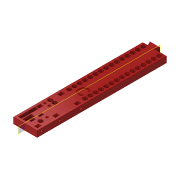
# Autodesk Inventor part: Coupler extension arm short
Saved by Autodesk Inventor 2020 (Build 240168000, 168)
## iProperties
Created: 2019-10-02
Part Number: Coupler extension arm short
Material: Generic
Document SubType Name: Modeling
Designer: ball
Density: 1 g/cm^3
Appearance: Default
Author: ball
Autodesk Inventor part; units mm, degrees
ref_plane "YZ Plane" through (0, 0, 0) normal (1, 0, 0) x (0, 1, 0)
ref_plane "XZ Plane" through (0, 0, 0) normal (0, 1, 0) x (-1, 0, 0)
ref_plane "XY Plane" through (0, 0, 0) normal (0, 0, 1) x (1, 0, 0)
sketch "Sketch1" plane through (0, 0, 0) normal (0, 1, 0) x (-1, 0, 0)
  line L0 (0, 0) -> (35.5, 0)
  line L1 (35.5, 0) -> (35.5, -195)
  line L2 (35.5, -195) -> (0, -195)
  line L3 (0, -195) -> (0, 0)
  dimension "d0" = 35.5
  dimension "d1" = 195
  constraints: 8 end point, 2 parallel, 1 horizontal, 1 perpendicular
  measures "d0" distance of L1.end L2.end
  measures "d1" distance of L0.end L1.end
extrude "BlockShape" add sketch "Sketch1" along normal blind 9
sketch "Sketch3" plane through (0, 0, 0) normal (0, -1, 0) x (1, 0, 0)
  circle A0 centre (-10, -25) radius 3.25 construction
  line L0 (0, 0) -> (-35.5, 0) projected
  line L1 (-35.5, 0) -> (-35.5, -195) projected
  line L2 (-11.6286, -27.8125) -> (-13.25, -24.9958)
  line L3 (-13.25, -24.9958) -> (-11.6214, -22.1833)
  line L4 (-11.6214, -22.1833) -> (-8.3714, -22.1875)
  line L5 (-8.3714, -22.1875) -> (-6.75, -25.0042)
  line L6 (-6.75, -25.0042) -> (-8.3786, -27.8167)
  line L7 (-8.3786, -27.8167) -> (-11.6286, -27.8125)
  line L8 (0, -195) -> (0, 0) projected
  dimension "d15" = 6.5
  dimension "d16" = 25
  dimension "d26" = 10
  constraints: 12 end point, 1 coincident, 16 other
  measures "d16" distance from line of L0 point (-10, -25)
  measures "d26" distance from line of L8 point (-10, -25)
extrude "SlideMountingNutWell1" cut sketch "Sketch3" against normal blind 5
sketch "Sketch5" plane through (0, 9, 0) normal (0, 1, 0) x (1, 0, 0)
  line L0 (0, 0) -> (0, 195) projected
  line L1 (-35.5, 0) -> (0, 0) projected
  circle A0 centre (-10, 25) radius 1.7
  circle A1 centre (-10, 15) radius 1.7
  dimension "d36" = 3.4
  dimension "d37" = 25
  dimension "d137" = 3.4
  dimension "d138" = 15
  constraints: 2 centre point
  measures "d36" diameter of A0
  measures "d37" distance from line of L1 A0.centre
  measures "d137" diameter of A1
  measures "d138" distance from line of L1 A1.centre
extrude "SlideMountingHoles" cut sketch "Sketch5" against normal through all
sketch "Sketch6" plane through (0, 9, 0) normal (0, 1, 0) x (1, 0, 0)
  line L0 (-32.5, 4) -> (-27.7502, 4)
  line L1 (-27.7502, 4) -> (-27.7502, 29.4)
  line L2 (-27.7502, 29.4) -> (-32.5, 29.4)
  line L3 (-32.5, 29.4) -> (-32.5, 4)
  line L4 (-35.5, 0) -> (0, 0) projected
  line L5 (-35.5, 195) -> (-35.5, 0) projected
  line L6 (-25.7502, 4) -> (-21.0002, 4)
  line L7 (-21.0002, 4) -> (-21.0002, 16.7)
  line L8 (-21.0002, 16.7) -> (-25.7502, 16.7)
  line L9 (-25.7502, 16.7) -> (-25.7502, 4)
  line L10 (0, 0) -> (0, 195) construction
  line L11 (-35.5, 195) -> (0, 195) projected
  line L12 (0, 0) -> (-20, 0) construction
  line L13 (-20, 0) -> (-20, 195) construction
  line L14 (-20, 195) -> (0, 195) construction
  line L15 (0, 195) -> (0, 0)
  circle A0 centre (-23.3752, 41.7) radius 1.7
  circle A1 centre (-30.125, 41.7) radius 1.7
  circle A2 centre (-30.125, 49.7) radius 1.7
  circle A3 centre (-23.3752, 49.7) radius 1.7
  dimension "d43" = 4.7498
  dimension "d44" = 25.4
  dimension "d45" = 4
  dimension "d46" = 3
  dimension "d47" = 4.75
  dimension "d48" = 2
  dimension "d49" = 20
  dimension "d50" = 3.4
  dimension "d90" = 3.4
  dimension "d91" = 5.375
  dimension "d92" = 3.4
  dimension "d94" = 3.4
  dimension "d246" = 41.7
  dimension "d247" = 49.7
  dimension "d248" = 41.7
  dimension "d249" = 49.7
  constraints: 24 end point, 6 parallel, 4 centre point, 3 horizontal, 3 perpendicular, 1 point on line
  measures "d43" distance of L2.end L1.end
  measures "d44" distance of L1.end L0.end
  measures "d45" distance between parallel lines of L4 L0
  measures "d46" distance between parallel lines of L5 L3
  measures "d47" distance of L8.end L7.end
  measures "d48" distance between parallel lines of L9 L1
  measures "d49" distance of L13.end L14.end
  measures "d50" diameter of A0
  measures "d90" diameter of A1
  measures "d91" distance from line of L5 A1.centre
  measures "d92" diameter of A2
  measures "d94" diameter of A3
  measures "d246" distance from line of L4 A0.centre
  measures "d247" distance from line of L4 A3.centre
  measures "d248" distance from line of L4 A1.centre
  measures "d249" distance from line of L4 A2.centre
extrude "Shape" cut sketch "Sketch6" against normal through all contours L3 L2 L1 L0 | L9 L8 L7 L6 | A0 | A1 | A2 | A3
sketch "Sketch7" plane through (0, 0, 0) normal (0, -1, 0) x (1, 0, 0)
  circle A0 centre (-23.3752, -41.7) radius 1.7 projected
  circle A1 centre (-23.3752, -41.7) radius 3.25 construction
  line L0 (-23.3752, -38.45) -> (-20.5606, -40.075)
  line L1 (-20.5606, -40.075) -> (-20.5606, -43.325)
  line L2 (-20.5606, -43.325) -> (-23.3752, -44.95)
  line L3 (-23.3752, -44.95) -> (-26.1898, -43.325)
  line L4 (-26.1898, -43.325) -> (-26.1898, -40.075)
  line L5 (-26.1898, -40.075) -> (-23.3752, -38.45)
  line L6 (0, 0) -> (-35.5, 0) projected
  circle A2 centre (-30.125, -41.7) radius 3.25 construction
  line L7 (-35.5, 0) -> (-35.5, -195) projected
  line L8 (-30.1645, -44.9498) -> (-32.9591, -43.2907)
  line L9 (-32.9591, -43.2907) -> (-32.9196, -40.0409)
  line L10 (-32.9196, -40.0409) -> (-30.0855, -38.4502)
  line L11 (-30.0855, -38.4502) -> (-27.2909, -40.1093)
  line L12 (-27.2909, -40.1093) -> (-27.3304, -43.3591)
  line L13 (-27.3304, -43.3591) -> (-30.1645, -44.9498)
  dimension "d88" = 6.5
  dimension "d54" = 6.5
  dimension "d87" = 41.7
  dimension "d89" = 5.375
  constraints: 24 end point, 3 coincident, 1 centre point, 17 other
  measures "d54" diameter of A1
  measures "d87" distance from line of L6 A1.centre
  measures "d89" distance from line of L7 point (-30.125, -41.7)
extrude "TensionNutWells1" cut sketch "Sketch7" against normal blind 5
sketch "Sketch8" plane through (-35.5, 0, -195) normal (-1, 0, 0) x (0, 0, 1)
  circle A0 centre (184.65, 4.5) radius 1.4605
  line L0 (0, 9) -> (195, 9) projected
  line L1 (195, 0) -> (195, 9) projected
  circle A1 centre (171.95, 4.5) radius 1.4605
  dimension "d57" = 2.921
  dimension "d58" = 4.5
  dimension "d59" = 10.35
  dimension "d103" = 2.921
  dimension "d104" = 4.5
  dimension "d105" = 12.7
  constraints: 2 centre point
  measures "d57" diameter of A0
  measures "d58" distance from line of L0 A0.centre
  measures "d59" distance from line of L1 A0.centre
  measures "d103" diameter of A1
  measures "d104" distance from line of L0 A1.centre
  measures "d105" distance of A0.centre A1.centre
hole "PulleyMountingHoles" at (-35.5, 4.5, -10.35) at (-35.5, 4.5, -23.05) direction (1, 0, 0) diameter 2.921 depth 22.5 counterbore diameter 3.4 counterbore depth 1.5
sketch "Sketch9" plane through (-21.0002, 9, -16.7) normal (-1, 0, 0) x (0, 0, 1)
  circle A0 centre (6.35, -4.5) radius 1.4605 projected
  circle A1 centre (6.35, -4.5) radius 2.54
  point P0 (16.7, -9)
  dimension "d67" = 5.08
  constraints: 1 centre point, 1 coincident
  measures "d67" diameter of A1
extrude "PulleyStandoff1" add sketch "Sketch9" along normal blind 0.2032
sketch "Sketch10" plane through (-27.7502, 9, -29.4) normal (-1, 0, 0) x (0, 0, 1)
  circle A0 centre (6.35, -4.5) radius 1.7 projected
  circle A1 centre (6.35, -4.5) radius 2.54
  circle A2 centre (19.05, -4.5) radius 2.54 projected
  circle A3 centre (19.05, -4.5) radius 2.54
  circle A4 centre (19.05, -4.5) radius 1.7
  point P0 (29.4, -9)
  dimension "d70" = 5.08
  dimension "d106" = 3.4
  constraints: 3 centre point, 3 coincident
  measures "d70" diameter of A1
  measures "d106" diameter of A4
extrude "PulleyStandoff3" add sketch "Sketch10" along normal blind 0.2032
sketch "Sketch11" plane through (-25.7502, 9, -4) normal (1, 0, 0) x (0, 0, -1)
  circle A0 centre (6.35, -4.5) radius 1.7 projected
  circle A1 centre (6.35, -4.5) radius 2.54
  point P0 (-4, -9)
  dimension "d73" = 5.08
  constraints: 1 centre point, 1 coincident
  measures "d73" diameter of A1
extrude "PulleyStandoff2" add sketch "Sketch11" along normal blind 0.2032
sketch "Sketch12" plane through (-32.5, 9, -4) normal (1, 0, 0) x (0, 0, -1)
  circle A0 centre (6.35, -4.5) radius 1.7 projected
  circle A1 centre (6.35, -4.5) radius 2.54
  circle A2 centre (19.05, -4.5) radius 1.4605 projected
  circle A3 centre (19.05, -4.5) radius 2.54
  circle A4 centre (19.05, -4.5) radius 1.7
  point P0 (-4, -9)
  dimension "d76" = 5.08
  dimension "d107" = 5.08
  dimension "d108" = 3.4
  constraints: 3 centre point, 3 coincident
  measures "d76" diameter of A1
  measures "d107" diameter of A3
  measures "d108" diameter of A4
extrude "PulleyStandof4" add sketch "Sketch12" along normal blind 0.2032 contours A1 | A3
sketch "Sketch14" plane through (0, 0, -195) normal (0, 0, -1) x (-1, 0, 0)
  circle A0 centre (18, 4.5) radius 2.25
  line L0 (35.5, 0) -> (0, 0) projected
  line L1 (0, 0) -> (0, 9) projected
  dimension "d82" = 4.5
  dimension "d83" = 4.5
  dimension "d84" = 18
  constraints: 1 centre point
  measures "d82" diameter of A0
  measures "d83" distance from line of L0 A0.centre
  measures "d84" distance from line of L1 A0.centre
extrude "4mmShaft" cut sketch "Sketch14" against normal blind 41
sketch "Sketch15" plane through (0, 9, 0) normal (0, 1, 0) x (1, 0, 0)
  circle A0 centre (-30.125, 49.7) radius 1.7 projected
  circle A1 centre (-30.125, 49.7) radius 3.25 construction
  circle A2 centre (-23.3752, 49.7) radius 1.7 projected
  circle A3 centre (-23.3752, 49.7) radius 3.25 construction
  line L0 (-30.125, 52.95) -> (-27.3104, 51.325)
  line L1 (-27.3104, 51.325) -> (-27.3104, 48.075)
  line L2 (-27.3104, 48.075) -> (-30.125, 46.45)
  line L3 (-30.125, 46.45) -> (-32.9396, 48.075)
  line L4 (-32.9396, 48.075) -> (-32.9396, 51.325)
  line L5 (-32.9396, 51.325) -> (-30.125, 52.95)
  line L6 (-23.3752, 52.95) -> (-20.5606, 51.325)
  line L7 (-20.5606, 51.325) -> (-20.5606, 48.075)
  line L8 (-20.5606, 48.075) -> (-23.3752, 46.45)
  line L9 (-23.3752, 46.45) -> (-26.1898, 48.075)
  line L10 (-26.1898, 48.075) -> (-26.1898, 51.325)
  line L11 (-26.1898, 51.325) -> (-23.3752, 52.95)
  point P0 (0, 0)
  dimension "d95" = 6.5
  dimension "d96" = 6.5
  constraints: 24 end point, 4 coincident, 2 vertical alignment, 30 other
extrude "TensionNutWells2" cut sketch "Sketch15" against normal blind 5
ref_plane "PulleyMidPlane1" through (-30.1251, 9, -4) normal (1, 0, 0) x (0, 0, -1)
ref_plane "PulleyMidPlane2" through (-23.3752, 9, -4) normal (1, 0, 0) x (0, 0, -1)
sketch "Sketch26" plane through (-35.5, 0, -195) normal (-1, 0, 0) x (0, 0, 1)
  line L0 (165.6, 9) -> (165.6, 0) construction
  line L1 (156.5498, 0) -> (156.5498, 5) construction
  line L2 (138.824, 0) -> (135.776, 0) construction
  line L3 (5.524, 0) -> (2.476, 0) construction
  circle A0 centre (161.0749, 4.5) radius 1.45 construction
  circle A1 centre (103.213, 4.5) radius 1.45 construction
  line L4 (135.776, 9) -> (135.776, 0) construction
  line L5 (5.524, 9) -> (5.524, 0) construction
  line L6 (0, 9) -> (195, 9) projected
  circle A2 centre (70.65, 4.5) radius 1.45 construction
  circle A3 centre (38.087, 4.5) radius 1.45 construction
  point P0 (195, 0)
  dimension "d192" = 2.9
  dimension "d193" = 2.9
  dimension "d196" = 130.252
  dimension "d197" = 32.563
  dimension "d198" = 4.5
  dimension "d199" = 4.5
  dimension "d202" = 32.563
  dimension "d207" = 9.0502
  dimension "d208" = 4.5251
  constraints: 4 centre point, 3 coincident, 1 horizontal, 4 other
  measures "d192" diameter of A0
  measures "d193" diameter of A1
  measures "d196" distance between parallel lines of L5 L4
  measures "d197" distance from line of L4 A1.centre
  measures "d198" distance from line of L6 A0.centre
  measures "d199" distance from line of L6 A1.centre
  measures "d202" distance of A1.centre A2.centre
  measures "d207" distance between parallel lines of L1 L0
  measures "d208" distance from line of L0 A0.centre
ref_plane "Work Plane3" through (-7.7, 0, 0) normal (1, 0, 0) x (0, 0, -1)
sketch "Sketch27" plane through (-7.7, 0, 0) normal (1, 0, 0) x (0, 0, -1)
  line L0 (195, 9) -> (0, 9) projected
  line L1 (0, 0) -> (0, 9) projected
  circle A0 centre (6.65, 4.5) radius 3.45 construction
  line L2 (6.65, 1.05) -> (3.6622, 2.775)
  line L3 (3.6622, 2.775) -> (3.6622, 9)
  line L4 (9.6378, 9) -> (9.6378, 2.775)
  line L5 (9.6378, 2.775) -> (6.65, 1.05)
  line L6 (3.6622, 9) -> (9.6378, 9)
  circle A1 centre (33.9251, 4.5) radius 3.45 construction
  line L7 (33.9251, 1.05) -> (30.9373, 2.775)
  line L8 (30.9373, 2.775) -> (30.9373, 9)
  line L9 (36.9129, 9) -> (36.9129, 2.775)
  line L10 (36.9129, 2.775) -> (33.9251, 1.05)
  line L11 (30.9373, 9) -> (36.9129, 9)
  circle A2 centre (66, 4.5) radius 3.45 construction
  line L12 (66, 1.05) -> (63.0122, 2.775)
  line L13 (63.0122, 2.775) -> (63.0122, 9)
  line L14 (68.9878, 9) -> (68.9878, 2.775)
  line L15 (68.9878, 2.775) -> (66, 1.05)
  line L16 (63.0122, 9) -> (68.9878, 9)
  dimension "d218" = 6.9
  dimension "d283" = 6.9
  dimension "d288" = 6.9
  dimension "d216" = 4.5
  dimension "d217" = 6.65
  dimension "d281" = 33.9251
  dimension "d282" = 4.5
  dimension "d287" = 66
  constraints: 30 end point, 6 coincident, 3 vertical alignment, 2 point on line, 1 collinear, 24 other
  measures "d216" distance from line of L0 point (6.65, 4.5)
  measures "d217" distance from line of L1 point (6.65, 4.5)
  measures "d281" distance from line of L1 point (33.925, 4.5)
  measures "d282" distance from line of L0 point (33.925, 4.5)
  measures "d287" distance from line of L1 point (66, 4.5)
extrude "SideNutWell" cut sketch "Sketch27" along normal blind 4.4
sketch "Sketch28" plane through (0, 0, 0) normal (1, 0, 0) x (0, 0, -1)
  line L0 (9.6378, 2.775) -> (9.6378, 9) construction
  line L1 (3.6622, 9) -> (3.6622, 2.775) construction
  line L2 (3.6622, 2.775) -> (6.65, 1.05) construction
  line L3 (6.65, 1.05) -> (9.6378, 2.775) construction
  circle A0 centre (6.65, 4.5) radius 1.7
  line L4 (195, 0) -> (0, 0) projected
  circle A1 centre (66, 4.5) radius 1.7
  line L5 (0, 0) -> (0, 9) projected
  circle A2 centre (33.9251, 4.5) radius 1.7
  dimension "d221" = 3.4
  dimension "d222" = 4.5
  dimension "d291" = 3.4
  dimension "d292" = 66
  dimension "d293" = 4.5
  dimension "d295" = 3.4
  dimension "d296" = 33.9251
  dimension "d297" = 4.5
  constraints: 3 centre point
  measures "d221" diameter of A0
  measures "d222" distance from line of L4 A0.centre
  measures "d291" diameter of A1
  measures "d292" distance from line of L5 A1.centre
  measures "d293" distance from line of L4 A1.centre
  measures "d295" diameter of A2
  measures "d296" distance from line of L5 A2.centre
  measures "d297" distance from line of L4 A2.centre
extrude "SideNetWellHole" cut sketch "Sketch28" against normal blind 8.4
ref_plane "Work Plane4" through (-27.8, 0, -195) normal (-1, 0, 0) x (0, 0, 1)
sketch "Sketch30" plane through (-27.8, 0, -195) normal (-1, 0, 0) x (0, 0, 1)
  circle A0 centre (161.0749, 4.5) radius 3.45 construction
  line L0 (165.6, 9) -> (165.6, 0) construction
  line L1 (164.445, 0) -> (155.555, 0) construction
  line L2 (161.0749, 1.05) -> (158.0871, 2.775)
  line L3 (158.0871, 2.775) -> (158.0871, 6.225)
  line L4 (164.0627, 6.225) -> (164.0627, 2.775)
  line L5 (164.0627, 2.775) -> (161.0749, 1.05)
  line L6 (164.0627, 6.225) -> (164.0627, 9)
  line L7 (195, 9) -> (0, 9) projected
  line L8 (158.0871, 6.225) -> (158.0871, 9)
  line L9 (158.0696, 9) -> (158.0696, 3.048) projected
  line L10 (158.0871, 9) -> (164.0627, 9)
  line L11 (195, 0) -> (195, 9) projected
  line L12 (0, 0) -> (195, 0) projected
  circle A1 centre (129, 4.5) radius 3.45 construction
  line L13 (129, 1.05) -> (126.0122, 2.775)
  line L14 (126.0122, 2.775) -> (126.0122, 6.225)
  line L15 (131.9878, 6.225) -> (131.9878, 2.775)
  line L16 (131.9878, 2.775) -> (129, 1.05)
  line L17 (131.9878, 6.225) -> (131.9878, 9)
  line L18 (126.0122, 6.225) -> (126.0122, 9)
  line L19 (126.0122, 9) -> (131.9878, 9)
  point P0 (158.0871, 9)
  point P1 (131.9878, 9)
  point P2 (126.0122, 9)
  dimension "d228" = 6.9
  dimension "d286" = 6.9
  dimension "d229" = 4.5251
  dimension "d230" = 4.5
  dimension "d280" = 33.9251
  dimension "d284" = 66
  dimension "d285" = 4.5
  constraints: 28 end point, 2 coincident, 2 perpendicular, 2 vertical, 2 vertical alignment, 1 parallel, 1 point on line, 20 other
  measures "d229" distance from line of L0 point (161.075, 4.5)
  measures "d230" distance from line of L1 point (161.075, 4.5)
  measures "d280" distance from line of L11 point (161.075, 4.5)
  measures "d284" distance from line of L11 point (129, 4.5)
  measures "d285" distance from line of L12 point (129, 4.5)
extrude "SideNutWell2" cut sketch "Sketch30" along normal blind 4.4
sketch "Sketch31" plane through (-35.5, 0, -195) normal (-1, 0, 0) x (0, 0, 1)
  circle A0 centre (161.0749, 4.5) radius 1.45 construction
  circle A1 centre (161.0749, 4.5) radius 1.7
  circle A2 centre (129, 4.5) radius 1.7
  line L0 (195, 0) -> (195, 9) projected
  dimension "d233" = 3.4
  dimension "d289" = 3.4
  dimension "d290" = 66
  dimension "d294" = 33.9251
  constraints: 2 centre point, 1 coincident
  measures "d233" diameter of A1
  measures "d289" diameter of A2
  measures "d290" distance from line of L0 A2.centre
  measures "d294" distance from line of L0 A0.centre
extrude "SideNutWellHole2" cut sketch "Sketch31" against normal blind 8.4
sketch "Sketch33" plane through (0, 0, 0) normal (0, -1, 0) x (1, 0, 0)
  line L0 (0, -195) -> (-35.5, -195) projected
  line L1 (-27.9958, -195) -> (-19.0042, -195)
  line L2 (-19.0042, -195) -> (-19.0042, -195.254)
  line L3 (-19.0042, -195.254) -> (-27.9958, -195.254) construction
  line L4 (-27.9958, -195.254) -> (-27.9958, -195)
  line L5 (-23.5, -195.254) -> (-23.5, -195) construction
  line L6 (-35.5, 0) -> (-35.5, -195) construction
  line L7 (-27.9958, -195.254) -> (-19.0042, -195.254) construction
  line L8 (-19.0042, -195.254) -> (-19.0042, -201.35) construction
  line L9 (-19.0042, -201.35) -> (-27.9958, -201.35)
  line L10 (-27.9958, -201.35) -> (-27.9958, -195.254) construction
  line L11 (-27.9958, -201.35) -> (-31.0438, -201.35)
  line L12 (-31.0438, -201.35) -> (-27.9958, -195.254)
  line L13 (-19.0042, -201.35) -> (-15.9562, -201.35)
  line L14 (-15.9562, -201.35) -> (-19.0042, -195.254)
  point P0 (0, 0)
  dimension "d237" = 8.9916
  dimension "d238" = 0.254
  dimension "d239" = 12
  dimension "d240" = 8.9916
  dimension "d241" = 6.096
  dimension "d242" = 3.048
  dimension "d243" = 3.048
  constraints: 26 end point, 5 parallel, 2 horizontal, 2 midpoint, 2 perpendicular, 2 point on line
  measures "d237" distance of L2.end L3.end
  measures "d238" distance of L1.end L2.end
  measures "d239" distance between parallel lines of L6 L5
  measures "d240" distance of L8.end L9.end
  measures "d241" distance between parallel lines of L3 L9
  measures "d242" distance from line of L11.end L10
  measures "d243" distance from line of L13.end L8
extrude "Extrusion22" add sketch "Sketch33" against normal up to surface (9 mm away)
sketch "Sketch34" plane through (0, 0, 0) normal (0, -1, 0) x (1, 0, 0)
  circle A0 centre (-5.75, -78) radius 2 construction
  circle A1 centre (-29.75, -78) radius 2 construction
  circle A2 centre (-5.75, -78) radius 1.7
  circle A3 centre (-29.75, -78) radius 1.7
  line L0 (0, -195) -> (0, 0) projected
  circle A4 centre (-5.75, -86) radius 1.7
  circle A5 centre (-29.75, -86) radius 1.7
  circle A6 centre (-5.75, -94) radius 1.7
  circle A7 centre (-29.75, -94) radius 1.7
  circle A8 centre (-5.75, -102) radius 1.7
  circle A9 centre (-29.75, -102) radius 1.7
  circle A10 centre (-5.75, -110) radius 1.7
  circle A11 centre (-29.75, -110) radius 1.7
  circle A12 centre (-5.75, -118) radius 1.7
  circle A13 centre (-29.75, -118) radius 1.7
  circle A14 centre (-5.75, -126) radius 1.7
  circle A15 centre (-29.75, -126) radius 1.7
  circle A16 centre (-5.75, -134) radius 1.7
  circle A17 centre (-29.75, -134) radius 1.7
  circle A18 centre (-5.75, -142) radius 1.7
  circle A19 centre (-29.75, -142) radius 1.7
  circle A20 centre (-5.75, -150) radius 1.7
  circle A21 centre (-29.75, -150) radius 1.7
  circle A22 centre (-5.75, -158) radius 1.7
  circle A23 centre (-29.75, -158) radius 1.7
  circle A24 centre (-5.75, -166) radius 1.7
  circle A25 centre (-29.75, -166) radius 1.7
  circle A26 centre (-5.75, -174) radius 1.7
  circle A27 centre (-29.75, -174) radius 1.7
  circle A28 centre (-5.75, -182) radius 1.7
  circle A29 centre (-29.75, -182) radius 1.7
  circle A30 centre (-5.75, -190) radius 1.7
  circle A31 centre (-29.75, -190) radius 1.7
  dimension "d250" = 3.4
  dimension "d251" = 3.4
  dimension "d254" = 8
  constraints: 32 centre point, 2 coincident, 1 vertical, 60 other
  measures "d250" diameter of A2
  measures "d251" diameter of A3
  measures "d254" distance of A2.centre A4.centre
extrude "Extrusion23" cut sketch "Sketch34" against normal through all
sketch "Sketch35" plane through (0, 9, 0) normal (0, 1, 0) x (1, 0, 0)
  circle A0 centre (-29.75, 78) radius 1.7 construction
  circle A1 centre (-29.75, 78) radius 3.25 construction
  circle A2 centre (-5.75, 78) radius 1.7 construction
  circle A3 centre (-5.75, 78) radius 3.25 construction
  line L0 (-26.5, 78) -> (-28.125, 75.1854)
  line L1 (-28.125, 75.1854) -> (-31.375, 75.1854)
  line L2 (-31.375, 75.1854) -> (-33, 78)
  line L3 (-33, 78) -> (-31.375, 80.8146)
  line L4 (-31.375, 80.8146) -> (-28.125, 80.8146)
  line L5 (-28.125, 80.8146) -> (-26.5, 78)
  line L6 (-2.5, 78) -> (-4.125, 75.1854)
  line L7 (-4.125, 75.1854) -> (-7.375, 75.1854)
  line L8 (-7.375, 75.1854) -> (-9, 78)
  line L9 (-9, 78) -> (-7.375, 80.8146)
  line L10 (-7.375, 80.8146) -> (-4.125, 80.8146)
  line L11 (-4.125, 80.8146) -> (-2.5, 78)
  line L12 (-35.5, 195) -> (-35.5, 0) construction
  line L13 (-28.125, 83.1854) -> (-31.375, 83.1854)
  line L14 (-31.375, 83.1854) -> (-33, 86)
  line L15 (-26.5, 86) -> (-28.125, 83.1854)
  circle A4 centre (-29.75, 86) radius 3.25 construction
  line L16 (-33, 86) -> (-31.375, 88.8146)
  line L17 (-31.375, 88.8146) -> (-28.125, 88.8146)
  line L18 (-28.125, 88.8146) -> (-26.5, 86)
  line L19 (-7.375, 83.1854) -> (-9, 86)
  line L20 (-4.125, 83.1854) -> (-7.375, 83.1854)
  line L21 (-2.5, 86) -> (-4.125, 83.1854)
  line L22 (-9, 86) -> (-7.375, 88.8146)
  line L23 (-4.125, 88.8146) -> (-2.5, 86)
  circle A5 centre (-5.75, 86) radius 3.25 construction
  line L24 (-7.375, 88.8146) -> (-4.125, 88.8146)
  line L25 (-28.125, 91.1854) -> (-31.375, 91.1854)
  line L26 (-31.375, 91.1854) -> (-33, 94)
  line L27 (-26.5, 94) -> (-28.125, 91.1854)
  circle A6 centre (-29.75, 94) radius 3.25 construction
  line L28 (-33, 94) -> (-31.375, 96.8146)
  line L29 (-31.375, 96.8146) -> (-28.125, 96.8146)
  line L30 (-28.125, 96.8146) -> (-26.5, 94)
  line L31 (-7.375, 91.1854) -> (-9, 94)
  line L32 (-4.125, 91.1854) -> (-7.375, 91.1854)
  line L33 (-2.5, 94) -> (-4.125, 91.1854)
  line L34 (-9, 94) -> (-7.375, 96.8146)
  line L35 (-4.125, 96.8146) -> (-2.5, 94)
  circle A7 centre (-5.75, 94) radius 3.25 construction
  line L36 (-7.375, 96.8146) -> (-4.125, 96.8146)
  line L37 (-28.125, 99.1854) -> (-31.375, 99.1854)
  line L38 (-31.375, 99.1854) -> (-33, 102)
  line L39 (-26.5, 102) -> (-28.125, 99.1854)
  circle A8 centre (-29.75, 102) radius 3.25 construction
  line L40 (-33, 102) -> (-31.375, 104.8146)
  line L41 (-31.375, 104.8146) -> (-28.125, 104.8146)
  line L42 (-28.125, 104.8146) -> (-26.5, 102)
  line L43 (-7.375, 99.1854) -> (-9, 102)
  line L44 (-4.125, 99.1854) -> (-7.375, 99.1854)
  line L45 (-2.5, 102) -> (-4.125, 99.1854)
  line L46 (-9, 102) -> (-7.375, 104.8146)
  line L47 (-4.125, 104.8146) -> (-2.5, 102)
  circle A9 centre (-5.75, 102) radius 3.25 construction
  line L48 (-7.375, 104.8146) -> (-4.125, 104.8146)
  line L49 (-28.125, 107.1854) -> (-31.375, 107.1854)
  line L50 (-31.375, 107.1854) -> (-33, 110)
  line L51 (-26.5, 110) -> (-28.125, 107.1854)
  circle A10 centre (-29.75, 110) radius 3.25 construction
  line L52 (-33, 110) -> (-31.375, 112.8146)
  line L53 (-31.375, 112.8146) -> (-28.125, 112.8146)
  line L54 (-28.125, 112.8146) -> (-26.5, 110)
  line L55 (-7.375, 107.1854) -> (-9, 110)
  line L56 (-4.125, 107.1854) -> (-7.375, 107.1854)
  line L57 (-2.5, 110) -> (-4.125, 107.1854)
  line L58 (-9, 110) -> (-7.375, 112.8146)
  line L59 (-4.125, 112.8146) -> (-2.5, 110)
  circle A11 centre (-5.75, 110) radius 3.25 construction
  line L60 (-7.375, 112.8146) -> (-4.125, 112.8146)
  line L61 (-28.125, 115.1854) -> (-31.375, 115.1854)
  line L62 (-31.375, 115.1854) -> (-33, 118)
  line L63 (-26.5, 118) -> (-28.125, 115.1854)
  circle A12 centre (-29.75, 118) radius 3.25 construction
  line L64 (-33, 118) -> (-31.375, 120.8146)
  line L65 (-31.375, 120.8146) -> (-28.125, 120.8146)
  line L66 (-28.125, 120.8146) -> (-26.5, 118)
  line L67 (-7.375, 115.1854) -> (-9, 118)
  line L68 (-4.125, 115.1854) -> (-7.375, 115.1854)
  line L69 (-2.5, 118) -> (-4.125, 115.1854)
  line L70 (-9, 118) -> (-7.375, 120.8146)
  line L71 (-4.125, 120.8146) -> (-2.5, 118)
  circle A13 centre (-5.75, 118) radius 3.25 construction
  line L72 (-7.375, 120.8146) -> (-4.125, 120.8146)
  line L73 (-28.125, 123.1854) -> (-31.375, 123.1854)
  line L74 (-31.375, 123.1854) -> (-33, 126)
  line L75 (-26.5, 126) -> (-28.125, 123.1854)
  circle A14 centre (-29.75, 126) radius 3.25 construction
  line L76 (-33, 126) -> (-31.375, 128.8146)
  line L77 (-31.375, 128.8146) -> (-28.125, 128.8146)
  line L78 (-28.125, 128.8146) -> (-26.5, 126)
  line L79 (-7.375, 123.1854) -> (-9, 126)
  line L80 (-4.125, 123.1854) -> (-7.375, 123.1854)
  line L81 (-2.5, 126) -> (-4.125, 123.1854)
  line L82 (-9, 126) -> (-7.375, 128.8146)
  line L83 (-4.125, 128.8146) -> (-2.5, 126)
  circle A15 centre (-5.75, 126) radius 3.25 construction
  line L84 (-7.375, 128.8146) -> (-4.125, 128.8146)
  line L85 (-28.125, 131.1854) -> (-31.375, 131.1854)
  line L86 (-31.375, 131.1854) -> (-33, 134)
  line L87 (-26.5, 134) -> (-28.125, 131.1854)
  circle A16 centre (-29.75, 134) radius 3.25 construction
  line L88 (-33, 134) -> (-31.375, 136.8146)
  line L89 (-31.375, 136.8146) -> (-28.125, 136.8146)
  line L90 (-28.125, 136.8146) -> (-26.5, 134)
  line L91 (-7.375, 131.1854) -> (-9, 134)
  line L92 (-4.125, 131.1854) -> (-7.375, 131.1854)
  line L93 (-2.5, 134) -> (-4.125, 131.1854)
  line L94 (-9, 134) -> (-7.375, 136.8146)
  line L95 (-4.125, 136.8146) -> (-2.5, 134)
  circle A17 centre (-5.75, 134) radius 3.25 construction
  line L96 (-7.375, 136.8146) -> (-4.125, 136.8146)
  line L97 (-28.125, 139.1854) -> (-31.375, 139.1854)
  line L98 (-31.375, 139.1854) -> (-33, 142)
  line L99 (-26.5, 142) -> (-28.125, 139.1854)
  circle A18 centre (-29.75, 142) radius 3.25 construction
  line L100 (-33, 142) -> (-31.375, 144.8146)
  line L101 (-31.375, 144.8146) -> (-28.125, 144.8146)
  line L102 (-28.125, 144.8146) -> (-26.5, 142)
  line L103 (-7.375, 139.1854) -> (-9, 142)
  line L104 (-4.125, 139.1854) -> (-7.375, 139.1854)
  line L105 (-2.5, 142) -> (-4.125, 139.1854)
  line L106 (-9, 142) -> (-7.375, 144.8146)
  line L107 (-4.125, 144.8146) -> (-2.5, 142)
  circle A19 centre (-5.75, 142) radius 3.25 construction
  line L108 (-7.375, 144.8146) -> (-4.125, 144.8146)
  line L109 (-28.125, 147.1854) -> (-31.375, 147.1854)
  line L110 (-31.375, 147.1854) -> (-33, 150)
  line L111 (-26.5, 150) -> (-28.125, 147.1854)
  circle A20 centre (-29.75, 150) radius 3.25 construction
  line L112 (-33, 150) -> (-31.375, 152.8146)
  line L113 (-31.375, 152.8146) -> (-28.125, 152.8146)
  line L114 (-28.125, 152.8146) -> (-26.5, 150)
  line L115 (-7.375, 147.1854) -> (-9, 150)
  line L116 (-4.125, 147.1854) -> (-7.375, 147.1854)
  line L117 (-2.5, 150) -> (-4.125, 147.1854)
  line L118 (-9, 150) -> (-7.375, 152.8146)
  line L119 (-4.125, 152.8146) -> (-2.5, 150)
  circle A21 centre (-5.75, 150) radius 3.25 construction
  line L120 (-7.375, 152.8146) -> (-4.125, 152.8146)
  line L121 (-28.125, 155.1854) -> (-31.375, 155.1854)
  line L122 (-31.375, 155.1854) -> (-33, 158)
  line L123 (-26.5, 158) -> (-28.125, 155.1854)
  circle A22 centre (-29.75, 158) radius 3.25 construction
  line L124 (-33, 158) -> (-31.375, 160.8146)
  line L125 (-31.375, 160.8146) -> (-28.125, 160.8146)
  line L126 (-28.125, 160.8146) -> (-26.5, 158)
  line L127 (-7.375, 155.1854) -> (-9, 158)
  line L128 (-4.125, 155.1854) -> (-7.375, 155.1854)
  line L129 (-2.5, 158) -> (-4.125, 155.1854)
  line L130 (-9, 158) -> (-7.375, 160.8146)
  line L131 (-4.125, 160.8146) -> (-2.5, 158)
  circle A23 centre (-5.75, 158) radius 3.25 construction
  line L132 (-7.375, 160.8146) -> (-4.125, 160.8146)
  line L133 (-28.125, 163.1854) -> (-31.375, 163.1854)
  line L134 (-31.375, 163.1854) -> (-33, 166)
  line L135 (-26.5, 166) -> (-28.125, 163.1854)
  circle A24 centre (-29.75, 166) radius 3.25 construction
  line L136 (-33, 166) -> (-31.375, 168.8146)
  line L137 (-31.375, 168.8146) -> (-28.125, 168.8146)
  line L138 (-28.125, 168.8146) -> (-26.5, 166)
  line L139 (-7.375, 163.1854) -> (-9, 166)
  line L140 (-4.125, 163.1854) -> (-7.375, 163.1854)
  line L141 (-2.5, 166) -> (-4.125, 163.1854)
  line L142 (-9, 166) -> (-7.375, 168.8146)
  line L143 (-4.125, 168.8146) -> (-2.5, 166)
  circle A25 centre (-5.75, 166) radius 3.25 construction
  line L144 (-7.375, 168.8146) -> (-4.125, 168.8146)
  line L145 (-28.125, 171.1854) -> (-31.375, 171.1854)
  line L146 (-31.375, 171.1854) -> (-33, 174)
  line L147 (-26.5, 174) -> (-28.125, 171.1854)
  circle A26 centre (-29.75, 174) radius 3.25 construction
  line L148 (-33, 174) -> (-31.375, 176.8146)
  line L149 (-31.375, 176.8146) -> (-28.125, 176.8146)
  line L150 (-28.125, 176.8146) -> (-26.5, 174)
  line L151 (-7.375, 171.1854) -> (-9, 174)
  line L152 (-4.125, 171.1854) -> (-7.375, 171.1854)
  line L153 (-2.5, 174) -> (-4.125, 171.1854)
  line L154 (-9, 174) -> (-7.375, 176.8146)
  line L155 (-4.125, 176.8146) -> (-2.5, 174)
  circle A27 centre (-5.75, 174) radius 3.25 construction
  line L156 (-7.375, 176.8146) -> (-4.125, 176.8146)
  line L157 (-28.125, 179.1854) -> (-31.375, 179.1854)
  line L158 (-31.375, 179.1854) -> (-33, 182)
  line L159 (-26.5, 182) -> (-28.125, 179.1854)
  circle A28 centre (-29.75, 182) radius 3.25 construction
  line L160 (-33, 182) -> (-31.375, 184.8146)
  line L161 (-31.375, 184.8146) -> (-28.125, 184.8146)
  line L162 (-28.125, 184.8146) -> (-26.5, 182)
  line L163 (-7.375, 179.1854) -> (-9, 182)
  line L164 (-4.125, 179.1854) -> (-7.375, 179.1854)
  line L165 (-2.5, 182) -> (-4.125, 179.1854)
  line L166 (-9, 182) -> (-7.375, 184.8146)
  line L167 (-4.125, 184.8146) -> (-2.5, 182)
  circle A29 centre (-5.75, 182) radius 3.25 construction
  line L168 (-7.375, 184.8146) -> (-4.125, 184.8146)
  line L169 (-28.125, 187.1854) -> (-31.375, 187.1854)
  line L170 (-31.375, 187.1854) -> (-33, 190)
  line L171 (-26.5, 190) -> (-28.125, 187.1854)
  circle A30 centre (-29.75, 190) radius 3.25 construction
  line L172 (-33, 190) -> (-31.375, 192.8146)
  line L173 (-31.375, 192.8146) -> (-28.125, 192.8146)
  line L174 (-28.125, 192.8146) -> (-26.5, 190)
  line L175 (-7.375, 187.1854) -> (-9, 190)
  line L176 (-4.125, 187.1854) -> (-7.375, 187.1854)
  line L177 (-2.5, 190) -> (-4.125, 187.1854)
  line L178 (-9, 190) -> (-7.375, 192.8146)
  line L179 (-4.125, 192.8146) -> (-2.5, 190)
  circle A31 centre (-5.75, 190) radius 3.25 construction
  line L180 (-7.375, 192.8146) -> (-4.125, 192.8146)
  point P0 (0, 0)
  dimension "d261" = 6.5
  dimension "d262" = 6.5
  dimension "d265" = 8
  constraints: 360 end point, 60 coincident, 30 horizontal alignment, 29 vertical, 506 other
  measures "d265" distance of point (-29.75, 78) point (-29.75, 86)
extrude "Extrusion24" cut sketch "Sketch35" against normal blind 5
ref_plane "Work Plane6" through (-19, 0, -195) normal (-1, 0, 0) x (0, 0, 1)
sketch "Sketch36" plane through (-19, 0, -195) normal (-1, 0, 0) x (0, 0, 1)
  circle A0 centre (171.95, 4.5) radius 1.4605 construction
  circle A1 centre (171.95, 4.5) radius 3.45 construction
  circle A2 centre (184.65, 4.5) radius 1.4605 construction
  circle A3 centre (184.65, 4.5) radius 3.45 construction
  line L0 (184.65, 1.05) -> (181.6622, 2.775)
  line L1 (181.6622, 2.775) -> (181.6622, 9)
  line L2 (187.6378, 9) -> (187.6378, 2.775)
  line L3 (187.6378, 2.775) -> (184.65, 1.05)
  line L4 (171.95, 1.05) -> (168.9622, 2.775)
  line L5 (168.9622, 2.775) -> (168.9622, 9)
  line L6 (174.9378, 9) -> (174.9378, 2.775)
  line L7 (174.9378, 2.775) -> (171.95, 1.05)
  line L8 (195, 9) -> (0, 9) projected
  line L9 (168.9622, 9) -> (174.9378, 9)
  line L10 (181.6622, 9) -> (187.6378, 9)
  point P0 (195, 0)
  dimension "d273" = 6.9
  dimension "d274" = 6.9
  constraints: 20 end point, 4 coincident, 4 point on line, 2 vertical alignment, 16 other
extrude "Extrusion25" cut sketch "Sketch36" against normal blind 2.8
sketch "Sketch37" plane through (0, 9, 0) normal (0, 1, 0) x (1, 0, 0)
  circle A0 centre (-10, 15) radius 1.7 projected
  circle A1 centre (-10, 15) radius 3.25 construction
  line L0 (-13.3066, 15) -> (-11.6533, 17.8636)
  line L1 (-11.6533, 17.8636) -> (-8.3467, 17.8636)
  line L2 (-8.3467, 17.8636) -> (-6.6934, 15)
  line L3 (-6.6934, 15) -> (-8.3467, 12.1364)
  line L4 (-8.3467, 12.1364) -> (-11.6533, 12.1364)
  line L5 (-11.6533, 12.1364) -> (-13.3066, 15)
  point P0 (0, 0)
  dimension "d277" = 6.5
  constraints: 12 end point, 2 coincident, 1 centre point, 13 other
  measures "d277" diameter of A1
extrude "Extrusion26" cut sketch "Sketch37" against normal blind 5
sketch "Sketch38" plane through (0, 9, 0) normal (0, 1, 0) x (1, 0, 0)
  line L0 (-25.4987, 95.3522) -> (-9.8566, 95.3522) construction
  line L1 (-9.8566, 95.3522) -> (-9.8566, 76.2818) construction
  line L2 (-9.8566, 76.2818) -> (-25.4987, 76.2818) construction
  line L3 (-25.4987, 76.2818) -> (-25.4987, 95.3522) construction
  spline S0 degree 2 poles (-16.2271, 77.9726) (-17.783, 77.9726) (-20.36, 78.9288) (-21.2838, 79.9013) knots 0 0 0 1 2 2 2
  spline S1 degree 2 poles (-21.2838, 79.9013) (-22.2076, 80.8575) (-23.2287, 83.8073) (-23.2287, 85.7846) knots 0 0 0 1 2 2 2
  spline S2 degree 2 poles (-23.2287, 85.7846) (-23.2287, 87.7619) (-22.1752, 90.6468) (-21.2838, 91.6192) knots 0 0 0 1 2 2 2
  spline S3 degree 2 poles (-21.2838, 91.6192) (-20.3924, 92.6079) (-17.7506, 93.6614) (-16.2271, 93.6614) knots 0 0 0 1 2 2 2
  spline S4 degree 2 poles (-16.2271, 93.6614) (-14.9953, 93.6614) (-12.6939, 92.9645) (-11.8025, 92.5107) knots 0 0 0 1 2 2 2
  line L4 (-11.8025, 92.5107) -> (-11.8025, 89.6744)
  line L5 (-11.8025, 89.6744) -> (-11.9483, 89.6744)
  spline S5 degree 2 poles (-11.9483, 89.6744) (-12.2238, 89.9013) (-13.0666, 90.4847) (-13.6663, 90.7927) knots 0 0 0 1 2 2 2
  spline S6 degree 2 poles (-13.6663, 90.7927) (-14.2012, 91.052) (-15.6274, 91.4572) (-16.2757, 91.4572) knots 0 0 0 1 2 2 2
  spline S7 degree 2 poles (-16.2757, 91.4572) (-18.2368, 91.4572) (-20.6193, 88.4912) (-20.6193, 85.7846) knots 0 0 0 1 2 2 2
  spline S8 degree 2 poles (-20.6193, 85.7846) (-20.6193, 83.1427) (-18.3178, 80.1768) (-16.2757, 80.1768) knots 0 0 0 1 2 2 2
  spline S9 degree 2 poles (-16.2757, 80.1768) (-15.0439, 80.1768) (-12.8073, 81.1979) (-11.9483, 81.992) knots 0 0 0 1 2 2 2
  line L6 (-11.9483, 81.992) -> (-11.8025, 81.992)
  line L7 (-11.8025, 81.992) -> (-11.8025, 79.1557)
  spline S10 degree 2 poles (-11.8025, 79.1557) (-12.1752, 78.9774) (-13.3097, 78.475) (-13.7636, 78.3616) knots 0 0 0 1 2 2 2
  spline S11 degree 2 poles (-13.7636, 78.3616) (-14.4119, 78.1671) (-15.4329, 77.9726) (-16.2271, 77.9726) knots 0 0 0 1 2 2 2
  point P0 (0, 0)
  constraints: 2 other
emboss "Emboss1" sketch "Sketch38" operation cut depth 1 direction (0, -1, 0)
sketch "Sketch40" plane through (0, 0, 0) normal (0, -1, 0) x (1, 0, 0)
  line L0 (-24.7422, -137.382) -> (-10.3219, -137.382) construction
  line L1 (-10.3219, -137.382) -> (-10.3219, -157.0181) construction
  line L2 (-10.3219, -157.0181) -> (-24.7422, -157.0181) construction
  line L3 (-24.7422, -157.0181) -> (-24.7422, -137.382) construction
  spline S0 degree 2 poles (-16.0815, -155.0445) (-17.6374, -155.0445) (-20.2144, -154.0882) (-21.1382, -153.1158) knots 0 0 0 1 2 2 2
  spline S1 degree 2 poles (-21.1382, -153.1158) (-22.062, -152.1595) (-23.0831, -149.2098) (-23.0831, -147.2325) knots 0 0 0 1 2 2 2
  spline S2 degree 2 poles (-23.0831, -147.2325) (-23.0831, -145.2552) (-22.0296, -142.3702) (-21.1382, -141.3978) knots 0 0 0 1 2 2 2
  spline S3 degree 2 poles (-21.1382, -141.3978) (-20.2468, -140.4091) (-17.605, -139.3556) (-16.0815, -139.3556) knots 0 0 0 1 2 2 2
  spline S4 degree 2 poles (-16.0815, -139.3556) (-14.8497, -139.3556) (-12.5483, -140.0526) (-11.6568, -140.5064) knots 0 0 0 1 2 2 2
  line L4 (-11.6568, -140.5064) -> (-11.6568, -143.3427)
  line L5 (-11.6568, -143.3427) -> (-11.8027, -143.3427)
  spline S5 degree 2 poles (-11.8027, -143.3427) (-12.0782, -143.1158) (-12.921, -142.5323) (-13.5207, -142.2244) knots 0 0 0 1 2 2 2
  spline S6 degree 2 poles (-13.5207, -142.2244) (-14.0556, -141.965) (-15.4818, -141.5599) (-16.1301, -141.5599) knots 0 0 0 1 2 2 2
  spline S7 degree 2 poles (-16.1301, -141.5599) (-18.0912, -141.5599) (-20.4737, -144.5258) (-20.4737, -147.2325) knots 0 0 0 1 2 2 2
  spline S8 degree 2 poles (-20.4737, -147.2325) (-20.4737, -149.8743) (-18.1722, -152.8402) (-16.1301, -152.8402) knots 0 0 0 1 2 2 2
  spline S9 degree 2 poles (-16.1301, -152.8402) (-14.8983, -152.8402) (-12.6617, -151.8192) (-11.8027, -151.025) knots 0 0 0 1 2 2 2
  line L6 (-11.8027, -151.025) -> (-11.6568, -151.025)
  line L7 (-11.6568, -151.025) -> (-11.6568, -153.8613)
  spline S10 degree 2 poles (-11.6568, -153.8613) (-12.0296, -154.0396) (-13.1641, -154.542) (-13.6179, -154.6555) knots 0 0 0 1 2 2 2
  spline S11 degree 2 poles (-13.6179, -154.6555) (-14.2662, -154.85) (-15.2873, -155.0445) (-16.0815, -155.0445) knots 0 0 0 1 2 2 2
  point P0 (0, 0)
  constraints: 2 other
emboss "Emboss2" sketch "Sketch40" operation cut depth 1 direction (0, 1, 0)
equation "\"d197\" = 0.25 * d196"
equation "\"d198\" = d180"
equation "\"d199\" = d180"
equation "\"d202\" = d197"
equation "\"d208\" = 0.5 * d207"
equation "\"d229\" = 0.5 * d207"
equation "\"d240\" = d237"
equation "\"d243\" = d242"
equation "\"d180\" = 0.5 * d179"
equation "\"d179\" = 9"
body "Solid1"
